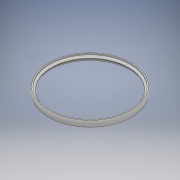
# Autodesk Inventor part: tyre
Saved by Autodesk Inventor 2018 (Build 220112000, 112)
## iProperties
Created: 2017-10-30
Part Number: tyre
Material: Generic
Document SubType Name: Modeling
Designer: erwin
Density: 1 g/cm^3
Appearance: Default
Author: erwin
Autodesk Inventor part; units mm, degrees
ref_plane "YZ Plane" through (0, 0, 0) normal (1, 0, 0) x (0, 1, 0)
ref_plane "XZ Plane" through (0, 0, 0) normal (0, 1, 0) x (-1, 0, 0)
ref_plane "XY Plane" through (0, 0, 0) normal (0, 0, 1) x (1, 0, 0)
sketch "Sketch2" plane through (0, 0, 0) normal (1, 0, 0) x (0, 1, 0)
  line L0 (41, 0.5464) -> (41, -0.4536)
  line L1 (41, -0.4536) -> (39, -2.4536)
  line L2 (39, -2.4536) -> (41, -4.4536)
  line L3 (41, 0.5464) -> (42, 0.5464)
  line L4 (42, -5.4536) -> (41, -5.4536)
  arc A0 (42, -5.4536) -> (42, 0.5464) centre (35.6754, -2.4536) ccw
  line L5 (41, -0.4536) -> (41, 0.5464)
  line L6 (0, 0.8214) -> (0, -16.8707) construction
  line L7 (41, -5.4536) -> (41, -4.4536)
  dimension "d2" = 41
  dimension "d5" = 6
  dimension "d6" = 1
  dimension "d8" = 1
  dimension "d9" = 7
  constraints: 16 end point, 3 equal length, 3 vertical, 2 perpendicular, 2 point on circle, 1 centre point, 1 collinear
  measures "d2" distance between parallel lines of L6 L0
  measures "d5" distance between parallel lines of L3 L4
  measures "d6" distance from line of L0.end L3
  measures "d8" distance of L0.start L3.end
  measures "d9" radius of A0
revolve "Revolution1" add sketch "Sketch2" angle 360 about axis through (0, 0, 0.8214) along (0, 0, -1)
fillet "Fillet1" radius 0.3 1 edges at (0, -39, -2.4536)
body "Solid1"
